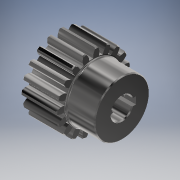
# Autodesk Inventor part: 歯車m2,z19
Saved by Autodesk Inventor 2019.2 (Build 232265000, 265)
## iProperties
Category: PARTsolutions
Company: KHK
Created: 2018-12-15
Part Number: 歯車m2,z19
Material: 鋼、高強度、低合金
Catalog Web Link: www.cadenas.de
Description: Ground Spur Gears (SSG)-
Vendor: KHK
Document SubType Name: Modeling
Designer: psadmin
Manufacturer: KHK
Mass: 35.2604 g
Surface Area: 82.0262 cm^2
Volume: 35.2604 cm^3
Density: 7.85 g/cm^3
Appearance: 鋼 - つや出し
PSOL_IDENT_0: {$CADENAS_DATA\23d-libs\khk\spur_gears\ground_spur_gears_ssg.prj},180 {VTYP=3D},{NB=SSG2-19J12},{LIN
PSOL_IDENT_1: A=SSG2-19J12},{NN=Ground Spur Gears (SSG)},{DATE=17.03.2017 04:28:20},{GEOMDATE=10.12.2014 11:17:00}
PSOL_IDENT_2: ,{VERSION=},{LINEID=23490},{WBVAR=},{WBNUMERIC=}  {NB=SSG2-19J12},{LINA=SSG2-19J12},{KT=DUMMY},{CN=S
PSOL_IDENT_3: SG2-19J12},{M=2.0},{Z=19},{A=12},{B=31},{C=38.0},{D=42.0},{E=20},{F=16},{G=36},{H=0},{I=0},{K=4},{KD=
PSOL_IDENT_4: 1.8},{M1=M4},{J=8.0},{S=S1K},{R=2},{N=1},{L=1},{L2=1},{X=3},{M11=4},{XX=4},{HIDE=0},{CBD1=0.0},{CBD2=
PSOL_IDENT_5: 0.0}
NN: Ground Spur Gears (SSG)
NB: SSG2-19J12
NBSYN: $CN.
LINA: SSG2-19J12
CN: SSG2-19J12
M: 2
Z: 19
A: 12
B: 31
C: 38
D: 42
E: 20
F: 16
G: 36
H: 0
I: 0
K: 4
KD: 1.8
M1: M4
J: 8
S: S1K
SUPPLIER: KHK
ARTICLENO: SSG2-19J12
BOMINFO: SSG2-19J12
CREATOR: CADENAS GmbH
Title: SSG2-19J12
Author: Cadenas PARTsolutions
Autodesk Inventor part; units mm, degrees
ref_plane "YZ Plane" through (0, 0, 0) normal (1, 0, 0) x (0, 1, 0)
ref_plane "XZ Plane" through (0, 0, 0) normal (0, 1, 0) x (-1, 0, 0)
ref_plane "XY Plane" through (0, 0, 0) normal (0, 0, 1) x (1, 0, 0)
sketch "Sketch_1" plane through (0, 0, 0) normal (0, 0, 1) x (1, 0, 0)
  line L0 (36, 0) -> (0, 0)
  line L1 (0, 6.5) -> (0.5, 6)
  line L2 (0.5, 6) -> (35.5, 6)
  line L3 (35.5, 6) -> (36, 6.5)
  line L4 (36, 6.5) -> (36, 15)
  line L5 (36, 15) -> (35.5, 15.5)
  line L6 (35.5, 15.5) -> (21, 15.5)
  arc A0 (20, 16.5) -> (21, 15.5) centre (21, 16.5) ccw
  line L7 (20, 16.5) -> (20, 20.5)
  line L8 (20, 20.5) -> (19.5, 21)
  line L9 (19.5, 21) -> (0.5, 21)
  line L10 (0.5, 21) -> (0, 20.5)
  line L11 (0, 20.5) -> (0, 6.5)
  constraints: 24 end point, 2 point on circle, 1 centre point
revolve "Revolution1" add sketch "Sketch_1" angle 360 about axis through (36, 0, 0) along (1, 0, 0)
sketch "Sketch_6" plane through (0, 0, 0) normal (1, 0, 0) x (0, 1, 0)
  line L0 (4.2, 2) -> (4.2, -2)
  line L1 (4.2, -2) -> (7.8, -2)
  line L2 (7.8, -2) -> (7.8, 2)
  line L3 (7.8, 2) -> (4.2, 2)
  constraints: 8 end point
extrude "Extrusion1" cut sketch "Sketch_6" along normal blind 38
sketch "Sketch_2" plane through (0, 0, 0) normal (0, 0, 1) x (1, 0, 0)
  line L0 (28, 0) -> (28, 21)
  line L1 (28, 21) -> (30, 21)
  line L2 (30, 21) -> (30, 15.5)
  line L3 (30, 15.5) -> (29.621, 15.121)
  line L4 (29.621, 15.121) -> (29.621, 8.179)
  line L5 (29.621, 8.179) -> (30, 7.8)
  line L6 (30, 7.8) -> (30, 0)
  line L7 (30, 0) -> (28, 0)
  line L8 (28, 0) -> (28, 21)
  constraints: 18 end point
revolve "Revolution2" cut sketch "Sketch_2" angle 360 about axis through (28, 0, 0) along (0, -1, 0)
thread "Thread1" size "M4x0.7" class "6H" standard "ISO Metric profile" full length
sketch "Sketch_5" plane through (0, 0, 0) normal (0, 1, 0) x (-1, 0, 0)
  line L0 (-28, 0) -> (-28, -21)
  line L1 (-28, -21) -> (-30, -21)
  line L2 (-30, -21) -> (-30, -15.5)
  line L3 (-30, -15.5) -> (-29.621, -15.121)
  line L4 (-29.621, -15.121) -> (-29.621, -6.379)
  line L5 (-29.621, -6.379) -> (-30, -6)
  line L6 (-30, -6) -> (-30, 0)
  line L7 (-30, 0) -> (-28, 0)
  line L8 (-28, 0) -> (-28, -21)
  constraints: 18 end point
revolve "Revolution3" cut sketch "Sketch_5" angle 360 about axis through (28, 0, 0) along (0, 0, 1)
thread "Thread2" size "M4x0.7" class "6H" standard "ISO Metric profile" full length
sketch "スケッチ5" plane through (0, 0, 0) normal (-1, 0, 0) x (0, 0, 1)
  arc A0 (1.2686, 18.1191) -> (1.209, 17.8132) centre (3.0704, 17.6093) ccw
  arc A1 (1.6365, 19.0772) -> (1.2686, 18.1191) centre (6.2514, 16.7555) ccw
  arc A2 (2.7756, 20.8158) -> (1.6365, 19.0772) centre (9.6798, 15.05) ccw
  arc A3 (-4.6834, 17.5493) -> (-4.6404, 17.2406) centre (-2.8137, 17.6522) ccw
  arc A4 (-4.6465, 18.575) -> (-4.6834, 17.5493) centre (0.4721, 17.8775) ccw
  arc A5 (-4.1337, 20.5891) -> (-4.6465, 18.575) centre (4.2686, 17.3775) ccw
  arc A6 (-10.1279, 15.0777) -> (-9.987, 14.7997) centre (-8.3929, 15.7821) ccw
  arc A7 (-10.426, 16.0598) -> (-10.1279, 15.0777) centre (-5.3582, 17.0621) ccw
  arc A8 (-10.595, 18.1314) -> (-10.426, 16.0598) centre (-1.6052, 17.822) ccw
  arc A9 (-14.4748, 10.9723) -> (-14.2513, 10.755) centre (-13.0626, 12.2018) ccw
  arc A10 (-15.0757, 11.8043) -> (-14.4748, 10.9723) centre (-10.608, 14.3978) ccw
  arc A11 (-15.9082, 13.7088) -> (-15.0757, 11.8043) centre (-7.305, 16.3351) ccw
  arc A12 (-17.2532, 5.6778) -> (-16.9713, 5.5449) centre (-16.3168, 7.2992) ccw
  arc A13 (-18.0917, 6.2697) -> (-17.2532, 5.6778) centre (-14.7082, 10.1733) ccw
  arc A14 (-19.4974, 7.8006) -> (-18.0917, 6.2697) centre (-12.2132, 13.0781) ccw
  arc A15 (-18.162, -0.232) -> (-17.8522, -0.2661) centre (-17.8027, 1.6057) ccw
  arc A16 (-19.1472, 0.0556) -> (-18.162, -0.232) centre (-17.2145, 4.8463) ccw
  arc A17 (-20.9739, 1.0471) -> (-19.1472, 0.0556) centre (-15.7979, 8.4039) ccw
  arc A18 (-17.1026, -6.1166) -> (-16.7985, -6.0483) centre (-17.3595, -4.2618) ccw
  arc A19 (-18.1278, -6.1645) -> (-17.1026, -6.1166) centre (-17.8554, -1.0058) ccw
  arc A20 (-20.1775, -5.8198) -> (-18.1278, -6.1645) centre (-17.6707, 2.819) ccw
  arc A21 (-14.1899, -11.3384) -> (-13.9244, -11.175) centre (-15.0351, -9.6675) ccw
  arc A22 (-15.144, -11.7166) -> (-14.1899, -11.3384) centre (-16.5614, -6.7489) ccw
  arc A23 (-17.1945, -12.0561) -> (-15.144, -11.7166) centre (-17.6286, -3.0714) ccw
  arc A24 (-9.7395, -15.3315) -> (-9.5414, -15.0908) centre (-11.0814, -14.0256) ccw
  arc A25 (-10.5191, -15.999) -> (-9.7395, -15.3315) centre (-13.4726, -11.7607) ccw
  arc A26 (-12.3483, -16.9859) -> (-10.5191, -15.999) centre (-15.6761, -8.629) ccw
  arc A27 (-4.2336, -17.6632) -> (-4.1245, -17.3712) centre (-5.9269, -16.8638) ccw
  arc A28 (-4.7542, -18.5477) -> (-4.2336, -17.6632) centre (-8.924, -15.498) ccw
  arc A29 (-6.1639, -20.075) -> (-4.7542, -18.5477) centre (-12.0249, -13.2515) ccw
  arc A30 (1.731, -18.0808) -> (1.7394, -17.7692) centre (-0.1301, -17.8745) ccw
  arc A31 (1.5258, -19.0864) -> (1.731, -18.0808) centre (-3.4082, -17.5559) ccw
  arc A32 (0.6884, -20.9887) -> (1.5258, -19.0864) centre (-7.0706, -16.4379) ccw
  arc A33 (7.508, -16.5391) -> (7.4148, -16.2417) centre (5.6808, -16.9483) ccw
  arc A34 (7.6405, -17.5568) -> (7.508, -16.5391) centre (2.4768, -17.7113) ccw
  arc A35 (7.4662, -19.6279) -> (7.6405, -17.5568) centre (-1.3501, -17.8431) ccw
  arc A36 (12.4714, -13.2051) -> (12.2867, -12.9541) centre (10.8761, -14.1854) ccw
  arc A37 (12.9272, -14.1247) -> (12.4714, -13.2051) centre (8.0935, -15.9475) ccw
  arc A38 (13.4348, -16.1402) -> (12.9272, -14.1247) centre (4.5167, -17.3147) ccw
  arc A39 (16.0834, -8.4401) -> (15.8272, -8.2627) centre (14.8928, -9.8853) ccw
  arc A40 (16.813, -9.1619) -> (16.0834, -8.4401) centre (12.8331, -12.4554) ccw
  arc A41 (17.9476, -10.9034) -> (16.813, -9.1619) centre (9.894, -14.91) ccw
  arc A42 (17.9525, -2.7606) -> (17.6525, -2.6759) centre (17.2956, -4.514) ccw
  arc A43 (18.8769, -3.2063) -> (17.9525, -2.7606) centre (16.182, -7.6137) ccw
  arc A44 (20.5155, -4.485) -> (18.8769, -3.2063) centre (14.1992, -10.8895) ccw
  arc A45 (17.8761, 3.2182) -> (17.5649, 3.2008) centre (17.8242, 1.3464) ccw
  arc A46 (18.8952, 3.0967) -> (17.8761, 3.2182) centre (17.7774, -1.9468) ccw
  arc A47 (20.8602, 2.4193) -> (18.8952, 3.0967) centre (16.9657, -5.689) ccw
  arc A48 (15.8626, 8.8482) -> (15.5739, 8.7307) centre (16.4213, 7.061) ccw
  arc A49 (16.8659, 9.0642) -> (15.8626, 8.8482) centre (17.4463, 3.931) ccw
  arc A50 (18.9444, 9.0615) -> (16.8659, 9.0642) centre (17.8937, 0.128) ccw
  arc A51 (12.1301, 13.5193) -> (11.8952, 13.3145) centre (13.2388, 12.0104) ccw
  arc A52 (13.0089, 14.0494) -> (12.1301, 13.5193) centre (15.2246, 9.3828) ccw
  arc A53 (14.9756, 14.7218) -> (13.0089, 14.0494) centre (16.8826, 5.9311) ccw
  arc A54 (7.0832, 16.7254) -> (6.9275, 16.4554) centre (8.6217, 15.6583) ccw
  arc A55 (7.7422, 17.5122) -> (7.0832, 16.7254) centre (11.3531, 13.8178) ccw
  arc A56 (9.3841, 18.7867) -> (7.7422, 17.5122) centre (14.042, 11.0915) ccw
  arc A57 (-1.209, 17.8132) -> (-1.2686, 18.1191) centre (-3.0704, 17.6093) ccw
  arc A58 (-1.2686, 18.1191) -> (-1.6365, 19.0772) centre (-6.2514, 16.7555) ccw
  arc A59 (-1.6365, 19.0772) -> (-2.7756, 20.8158) centre (-9.6798, 15.05) ccw
  arc A60 (-6.9275, 16.4554) -> (-7.0832, 16.7254) centre (-8.6217, 15.6583) ccw
  arc A61 (-7.0832, 16.7254) -> (-7.7422, 17.5122) centre (-11.3531, 13.8178) ccw
  arc A62 (-7.7422, 17.5122) -> (-9.3841, 18.7867) centre (-14.042, 11.0915) ccw
  arc A63 (-11.8952, 13.3145) -> (-12.1301, 13.5193) centre (-13.2388, 12.0104) ccw
  arc A64 (-12.1301, 13.5193) -> (-13.0089, 14.0494) centre (-15.2246, 9.3828) ccw
  arc A65 (-13.0089, 14.0494) -> (-14.9756, 14.7218) centre (-16.8826, 5.9311) ccw
  arc A66 (-15.5739, 8.7307) -> (-15.8626, 8.8482) centre (-16.4213, 7.061) ccw
  arc A67 (-15.8626, 8.8482) -> (-16.8659, 9.0642) centre (-17.4463, 3.931) ccw
  arc A68 (-16.8659, 9.0642) -> (-18.9444, 9.0615) centre (-17.8937, 0.128) ccw
  arc A69 (-17.5649, 3.2008) -> (-17.8761, 3.2182) centre (-17.8242, 1.3464) ccw
  arc A70 (-17.8761, 3.2182) -> (-18.8952, 3.0967) centre (-17.7774, -1.9468) ccw
  arc A71 (-18.8952, 3.0967) -> (-20.8602, 2.4193) centre (-16.9657, -5.689) ccw
  arc A72 (-17.6525, -2.6759) -> (-17.9525, -2.7606) centre (-17.2956, -4.514) ccw
  arc A73 (-17.9525, -2.7606) -> (-18.8769, -3.2063) centre (-16.182, -7.6137) ccw
  arc A74 (-18.8769, -3.2063) -> (-20.5155, -4.485) centre (-14.1992, -10.8895) ccw
  arc A75 (-15.8272, -8.2627) -> (-16.0834, -8.4401) centre (-14.8928, -9.8853) ccw
  arc A76 (-16.0834, -8.4401) -> (-16.813, -9.1619) centre (-12.8331, -12.4554) ccw
  arc A77 (-16.813, -9.1619) -> (-17.9476, -10.9034) centre (-9.894, -14.91) ccw
  arc A78 (-12.2867, -12.9541) -> (-12.4714, -13.2051) centre (-10.8761, -14.1854) ccw
  arc A79 (-12.4714, -13.2051) -> (-12.9272, -14.1247) centre (-8.0935, -15.9475) ccw
  arc A80 (-12.9272, -14.1247) -> (-13.4348, -16.1402) centre (-4.5167, -17.3147) ccw
  arc A81 (-7.4148, -16.2417) -> (-7.508, -16.5391) centre (-5.6808, -16.9483) ccw
  arc A82 (-7.508, -16.5391) -> (-7.6405, -17.5568) centre (-2.4768, -17.7113) ccw
  arc A83 (-7.6405, -17.5568) -> (-7.4662, -19.6279) centre (1.3501, -17.8431) ccw
  arc A84 (-1.7394, -17.7692) -> (-1.731, -18.0808) centre (0.1301, -17.8745) ccw
  arc A85 (-1.731, -18.0808) -> (-1.5258, -19.0864) centre (3.4082, -17.5559) ccw
  arc A86 (-1.5258, -19.0864) -> (-0.6884, -20.9887) centre (7.0706, -16.4379) ccw
  arc A87 (4.1245, -17.3712) -> (4.2336, -17.6632) centre (5.9269, -16.8638) ccw
  arc A88 (4.2336, -17.6632) -> (4.7542, -18.5477) centre (8.924, -15.498) ccw
  arc A89 (4.7542, -18.5477) -> (6.1639, -20.075) centre (12.0249, -13.2515) ccw
  arc A90 (9.5414, -15.0908) -> (9.7395, -15.3315) centre (11.0814, -14.0256) ccw
  arc A91 (9.7395, -15.3315) -> (10.5191, -15.999) centre (13.4726, -11.7607) ccw
  arc A92 (10.5191, -15.999) -> (12.3483, -16.9859) centre (15.6761, -8.629) ccw
  arc A93 (13.9244, -11.175) -> (14.1899, -11.3384) centre (15.0351, -9.6675) ccw
  arc A94 (14.1899, -11.3384) -> (15.144, -11.7166) centre (16.5614, -6.7489) ccw
  arc A95 (15.144, -11.7166) -> (17.1945, -12.0561) centre (17.6286, -3.0714) ccw
  arc A96 (16.7985, -6.0483) -> (17.1026, -6.1166) centre (17.3595, -4.2618) ccw
  arc A97 (17.1026, -6.1166) -> (18.1278, -6.1645) centre (17.8554, -1.0058) ccw
  arc A98 (18.1278, -6.1645) -> (20.1775, -5.8198) centre (17.6707, 2.819) ccw
  arc A99 (17.8522, -0.2661) -> (18.162, -0.232) centre (17.8027, 1.6057) ccw
  arc A100 (18.162, -0.232) -> (19.1472, 0.0556) centre (17.2145, 4.8463) ccw
  arc A101 (19.1472, 0.0556) -> (20.9739, 1.0471) centre (15.7979, 8.4039) ccw
  arc A102 (16.9713, 5.5449) -> (17.2532, 5.6778) centre (16.3168, 7.2992) ccw
  arc A103 (17.2532, 5.6778) -> (18.0917, 6.2697) centre (14.7082, 10.1733) ccw
  arc A104 (18.0917, 6.2697) -> (19.4974, 7.8006) centre (12.2132, 13.0781) ccw
  arc A105 (14.2513, 10.755) -> (14.4748, 10.9723) centre (13.0626, 12.2018) ccw
  arc A106 (14.4748, 10.9723) -> (15.0757, 11.8043) centre (10.608, 14.3978) ccw
  arc A107 (15.0757, 11.8043) -> (15.9082, 13.7088) centre (7.305, 16.3351) ccw
  arc A108 (9.987, 14.7997) -> (10.1279, 15.0777) centre (8.3929, 15.7821) ccw
  arc A109 (10.1279, 15.0777) -> (10.426, 16.0598) centre (5.3582, 17.0621) ccw
  arc A110 (10.426, 16.0598) -> (10.595, 18.1314) centre (1.6052, 17.822) ccw
  arc A111 (4.6404, 17.2406) -> (4.6834, 17.5493) centre (2.8137, 17.6522) ccw
  arc A112 (4.6834, 17.5493) -> (4.6465, 18.575) centre (-0.4721, 17.8775) ccw
  arc A113 (4.6465, 18.575) -> (4.1337, 20.5891) centre (-4.2686, 17.3775) ccw
  arc A114 (1.1173, 16.4621) -> (-1.1173, 16.4621) centre (0, 0) ccw
  arc A115 (-4.2884, 15.933) -> (-6.402, 15.2074) centre (0, 0) ccw
  arc A116 (-9.2295, 13.6772) -> (-10.993, 12.3046) centre (0, 0) ccw
  arc A117 (-13.1704, 9.9393) -> (-14.3927, 8.0685) centre (0, 0) ccw
  arc A118 (-15.6841, 5.1244) -> (-16.2327, 2.9581) centre (0, 0) ccw
  arc A119 (-16.4982, -0.2459) -> (-16.3136, -2.4729) centre (0, 0) ccw
  arc A120 (-15.5244, -5.5895) -> (-14.6267, -7.636) centre (0, 0) ccw
  arc A121 (-12.8683, -10.3274) -> (-11.3548, -11.9715) centre (0, 0) ccw
  arc A122 (-8.8178, -13.9462) -> (-6.8524, -15.0098) centre (0, 0) ccw
  arc A123 (-3.8117, -16.0537) -> (-1.6075, -16.4215) centre (0, 0) ccw
  arc A124 (1.6075, -16.4215) -> (3.8117, -16.0537) centre (0, 0) ccw
  arc A125 (6.8524, -15.0098) -> (8.8178, -13.9462) centre (0, 0) ccw
  arc A126 (11.3548, -11.9715) -> (12.8683, -10.3274) centre (0, 0) ccw
  arc A127 (14.6267, -7.636) -> (15.5244, -5.5895) centre (0, 0) ccw
  arc A128 (16.3136, -2.4729) -> (16.4982, -0.2459) centre (0, 0) ccw
  arc A129 (16.2327, 2.9581) -> (15.6841, 5.1244) centre (0, 0) ccw
  arc A130 (14.3927, 8.0685) -> (13.1704, 9.9393) centre (0, 0) ccw
  arc A131 (10.993, 12.3046) -> (9.2295, 13.6772) centre (0, 0) ccw
  arc A132 (6.402, 15.2074) -> (4.2884, 15.933) centre (0, 0) ccw
  arc A133 (-2.7756, 20.8158) -> (-4.1337, 20.5891) centre (0, 0) ccw
  arc A134 (-9.3841, 18.7867) -> (-10.595, 18.1314) centre (0, 0) ccw
  arc A135 (-14.9756, 14.7218) -> (-15.9082, 13.7088) centre (0, 0) ccw
  arc A136 (-18.9444, 9.0615) -> (-19.4974, 7.8006) centre (0, 0) ccw
  arc A137 (-20.8602, 2.4193) -> (-20.9739, 1.0471) centre (0, 0) ccw
  arc A138 (-20.5155, -4.485) -> (-20.1775, -5.8198) centre (0, 0) ccw
  arc A139 (-17.9476, -10.9034) -> (-17.1945, -12.0561) centre (0, 0) ccw
  arc A140 (-13.4348, -16.1402) -> (-12.3483, -16.9859) centre (0, 0) ccw
  arc A141 (-7.4662, -19.6279) -> (-6.1639, -20.075) centre (0, 0) ccw
  arc A142 (-0.6884, -20.9887) -> (0.6884, -20.9887) centre (0, 0) ccw
  arc A143 (6.1639, -20.075) -> (7.4662, -19.6279) centre (0, 0) ccw
  arc A144 (12.3483, -16.9859) -> (13.4348, -16.1402) centre (0, 0) ccw
  arc A145 (17.1945, -12.0561) -> (17.9476, -10.9034) centre (0, 0) ccw
  arc A146 (20.1775, -5.8198) -> (20.5155, -4.485) centre (0, 0) ccw
  arc A147 (20.9739, 1.0471) -> (20.8602, 2.4193) centre (0, 0) ccw
  arc A148 (19.4974, 7.8006) -> (18.9444, 9.0615) centre (0, 0) ccw
  arc A149 (15.9082, 13.7088) -> (14.9756, 14.7218) centre (0, 0) ccw
  arc A150 (10.595, 18.1314) -> (9.3841, 18.7867) centre (0, 0) ccw
  arc A151 (4.1337, 20.5891) -> (2.7756, 20.8158) centre (0, 0) ccw
  line L0 (1.1173, 16.4621) -> (1.209, 17.8132)
  line L1 (-4.2884, 15.933) -> (-4.6404, 17.2406)
  line L2 (-9.2295, 13.6772) -> (-9.987, 14.7997)
  line L3 (-13.1704, 9.9393) -> (-14.2513, 10.755)
  line L4 (-15.6841, 5.1244) -> (-16.9713, 5.5449)
  line L5 (-16.4982, -0.2459) -> (-17.8522, -0.2661)
  line L6 (-15.5244, -5.5895) -> (-16.7985, -6.0483)
  line L7 (-12.8683, -10.3274) -> (-13.9244, -11.175)
  line L8 (-8.8178, -13.9462) -> (-9.5414, -15.0908)
  line L9 (-3.8117, -16.0537) -> (-4.1245, -17.3712)
  line L10 (1.6075, -16.4215) -> (1.7394, -17.7692)
  line L11 (6.8524, -15.0098) -> (7.4148, -16.2417)
  line L12 (11.3548, -11.9715) -> (12.2867, -12.9541)
  line L13 (14.6267, -7.636) -> (15.8272, -8.2627)
  line L14 (16.3136, -2.4729) -> (17.6525, -2.6759)
  line L15 (16.2327, 2.9581) -> (17.5649, 3.2008)
  line L16 (14.3927, 8.0685) -> (15.5739, 8.7307)
  line L17 (10.993, 12.3046) -> (11.8952, 13.3145)
  line L18 (6.402, 15.2074) -> (6.9275, 16.4554)
  line L19 (-1.1173, 16.4621) -> (-1.209, 17.8132)
  line L20 (-6.402, 15.2074) -> (-6.9275, 16.4554)
  line L21 (-10.993, 12.3046) -> (-11.8952, 13.3145)
  line L22 (-14.3927, 8.0685) -> (-15.5739, 8.7307)
  line L23 (-16.2327, 2.9581) -> (-17.5649, 3.2008)
  line L24 (-16.3136, -2.4729) -> (-17.6525, -2.6759)
  line L25 (-14.6267, -7.636) -> (-15.8272, -8.2627)
  line L26 (-11.3548, -11.9715) -> (-12.2867, -12.9541)
  line L27 (-6.8524, -15.0098) -> (-7.4148, -16.2417)
  line L28 (-1.6075, -16.4215) -> (-1.7394, -17.7692)
  line L29 (3.8117, -16.0537) -> (4.1245, -17.3712)
  line L30 (8.8178, -13.9462) -> (9.5414, -15.0908)
  line L31 (12.8683, -10.3274) -> (13.9244, -11.175)
  line L32 (15.5244, -5.5895) -> (16.7985, -6.0483)
  line L33 (16.4982, -0.2459) -> (17.8522, -0.2661)
  line L34 (15.6841, 5.1244) -> (16.9713, 5.5449)
  line L35 (13.1704, 9.9393) -> (14.2513, 10.755)
  line L36 (9.2295, 13.6772) -> (9.987, 14.7997)
  line L37 (4.2884, 15.933) -> (4.6404, 17.2406)
  line L38 (-23, 0) -> (23, 0)
  line L39 (0, -23) -> (0, 23)
  line L40 (41, 21) -> (111, 21)
  line L41 (41, 13) -> (111, 13)
  line L42 (41, 5) -> (111, 5)
  line L43 (41, -3) -> (111, -3)
  line L44 (41, -11) -> (111, -11)
  line L45 (41, -19) -> (111, -19)
  line L46 (41, -27) -> (111, -27)
  line L47 (41, -35) -> (111, -35)
  line L48 (41, -43) -> (111, -43)
  line L49 (41, -51) -> (111, -51)
  line L50 (41, -59) -> (111, -59)
  line L51 (41, -67) -> (111, -67)
  line L52 (41, -75) -> (111, -75)
  line L53 (41, 21) -> (41, -75)
  line L54 (111, 21) -> (111, -75)
  line L55 (76, 13) -> (76, -75)
  circle A152 centre (0, 0) radius 21 projected
  point P0 (47, 15)
  point P1 (49.5, 7)
  point P2 (49.5, -1)
  point P3 (47, -9)
  point P4 (49.5, -17)
  point P5 (44.5, -25)
  point P6 (47, -33)
  point P7 (47, -41)
  point P8 (47, -49)
  point P9 (49.5, -57)
  point P10 (49.5, -65)
  point P11 (47, -73)
  point P12 (77, 7)
  point P13 (92, -1)
  point P14 (93.25, -9)
  point P15 (89.5, -17)
  point P16 (92, -25)
  point P17 (85.75, -33)
  point P18 (92, -41)
  point P19 (92, -49)
  point P20 (87, -57)
  point P21 (1, 36.5)
  point P22 (1, 30.5)
  point P23 (17.1875, 36.5)
  point P24 (19.3125, 30.5)
  constraints: 228 point on circle, 114 centre point, 108 end point, 2 horizontal alignment, 2 midpoint, 166 other
extrude "押し出し2" cut sketch "スケッチ5" against normal through all contours A0 L0 A114 L39 A152 A2 A1 | A114 L19 A57 A58 A59 A152 L39 | A152 A56 A55 A54 L18 A132 L37 A111 A112 A113 | L38 A152 A17 A16 | A16 A15 L5 A119 L24 A72 A73 A74 A152 L38 | L38 A152 A44 A43 A42 L14 A128 L33 A99 A100 | A100 A101 A152 L38 | A152 A53 A52 A51 L17 A131 L36 A108 A109 A110 | A5 A4 A3 L1 A115 L20 A60 A61 A62 A152 | A152 A29 A28 A27 L9 A123 L28 A84 A85 A86 | A32 A31 A30 L10 A124 L29 A87 A88 A89 A152 | A152 A50 A49 A48 L16 A130 L35 A105 A106 A107 | A8 A7 A6 L2 A116 L21 A63 A64 A65 A152 | A152 A14 A13 A12 L4 A118 L23 A69 A70 A71 | A20 A19 A18 L6 A120 L25 A75 A76 A77 A152 | A47 A46 A45 L15 A129 L34 A102 A103 A104 A152 | A152 A41 A40 A39 L13 A127 L32 A96 A97 A98 | A152 A26 A25 A24 L8 A122 L27 A81 A82 A83 | A35 A34 A33 L11 A125 L30 A90 A91 A92 A152 | A11 A10 A9 L3 A117 L22 A66 A67 A68 A152 | A23 A22 A21 L7 A121 L26 A78 A79 A80 A152 | A152 A38 A37 A36 L12 A126 L31 A93 A94 A95
body "Solid1"
